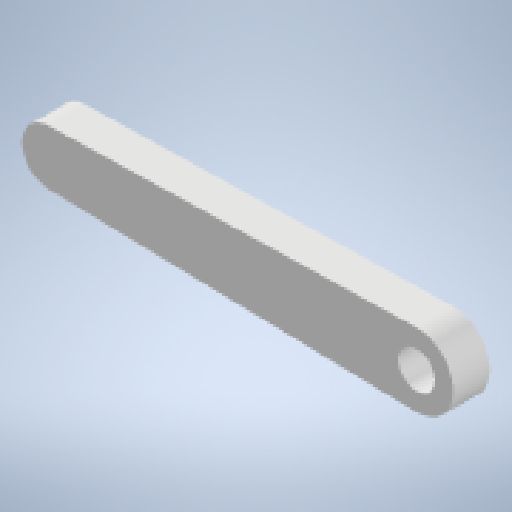
# Autodesk Inventor part: Brazo
Saved by Autodesk Inventor 2024 (Build 280153000, 153)
## iProperties
Created: 2023-08-25
Part Number: Brazo
Material: Genérico
Document SubType Name: Modeling
Designer: sergi
Density: 1 g/cm^3
Appearance: Valor por defecto
Author: sergi
Autodesk Inventor part; units mm, degrees
ref_plane "YZ Plane" through (0, 0, 0) normal (1, 0, 0) x (0, 1, 0)
ref_plane "XZ Plane" through (0, 0, 0) normal (0, 1, 0) x (-1, 0, 0)
ref_plane "XY Plane" through (0, 0, 0) normal (0, 0, 1) x (1, 0, 0)
sketch "Boceto1" plane through (0, 0, 0) normal (0, 0, 1) x (1, 0, 0)
  arc A0 (-0.1, -3.9987) -> (-0.1, 3.9987) centre (0, 0) ccw
  line L0 (0, 0) -> (-40, 0)
  arc A1 (-40.075, 2.9991) -> (-40.075, -2.9991) centre (-40, 0) ccw
  line L1 (-40.075, 2.9991) -> (-0.1, 3.9987)
  line L2 (-40.075, -2.9991) -> (-0.1, -3.9987)
  dimension "d0" = 8
  dimension "d1" = 40
  dimension "d2" = 6
  constraints: 6 end point, 4 point on circle, 4 tangent, 2 centre point, 2 coincident, 1 horizontal
  measures "d0" diameter of A0
  measures "d1" distance of L0.start L0.end
  measures "d2" diameter of A1
extrude "Extrusión1" add sketch "Boceto1" along normal blind 6
sketch "Boceto2" plane through (0, 0, 6) normal (0, 0, 1) x (1, 0, 0)
  arc A0 (-0.1, -3.9987) -> (-0.1, 3.9987) centre (0, 0) ccw projected
  constraints: 1 coincident
hole "Agujero1" at (0, 0, 6) direction (0, 0, -1) diameter 4 depth 11.75 tip angle 118
sketch "Boceto3" plane through (0, 0, 6) normal (0, 0, 1) x (1, 0, 0)
  line L0 (-1.5877, 2.75) -> (1.5877, 2.75)
  line L1 (1.5877, 2.75) -> (3.1754, 0)
  line L2 (3.1754, 0) -> (1.5877, -2.75)
  line L3 (1.5877, -2.75) -> (-1.5877, -2.75)
  line L4 (-1.5877, -2.75) -> (-3.1754, 0)
  line L5 (-3.1754, 0) -> (-1.5877, 2.75)
  point P0 (0, 0)
  point P1 (0, 0)
  dimension "d12" = 5.5
  constraints: 12 end point, 1 coincident, 1 horizontal, 13 other
  measures "d12" distance between parallel lines of L3 L0
extrude "Extrusión2" cut sketch "Boceto3" against normal blind 2
